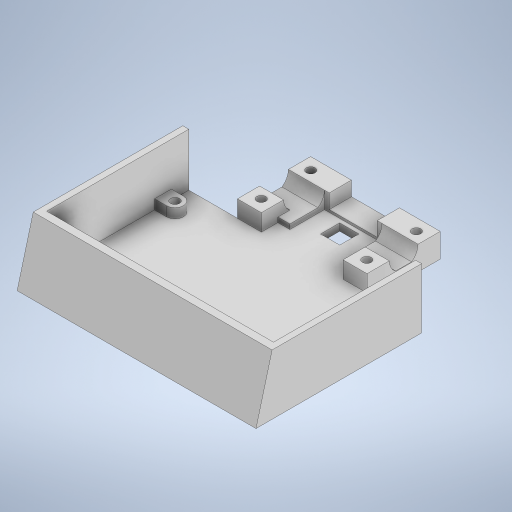
# Autodesk Inventor part: tělo estonsko s plechem otočené motory
Saved by Autodesk Inventor 2024 (Build 280153000, 153)
## iProperties
Created: 2023-09-06
Part Number: tělo estonsko s plechem otočené motory
Material: Všeobecné
Document SubType Name: Modeling
Designer: Simak
Density: 1 g/cm^3
Appearance: Výchozí
Author: Simak
Autodesk Inventor part; units mm, degrees
ref_plane "Pracovní rovina1" through (47.25, 44, 5) normal (0, 1, 0) x (1, 0, 0)
ref_plane "Pracovní rovina2" through (45.625, 37.275, -13.15) normal (0, 1, 0) x (1, 0, 0)
ref_plane "YZ Plane" through (0, 0, 0) normal (1, 0, 0) x (0, 1, 0)
sketch "Náčrt1" plane through (0, 0, 0) normal (0, 1, 0) x (-1, 0, 0)
  line L0 (49.75, -19.25) -> (49.75, 49.75)
  line L1 (49.75, 49.75) -> (-49.75, 49.75)
  line L2 (-49.75, 49.75) -> (-49.75, -19.25)
  line L3 (-49.75, -19.25) -> (-27, -19.25)
  line L4 (-27, -19.25) -> (-27, -49.75)
  line L5 (-27, -49.75) -> (27, -49.75)
  line L6 (27, -49.75) -> (27, -19.25)
  line L7 (27, -19.25) -> (49.75, -19.25)
  point P0 (0, 0)
  dimension "d0" = 30.5
  dimension "d1" = 99.5
  dimension "d2" = 22.75
  dimension "d3" = 99.5
  dimension "d4" = 54
  dimension "d5" = 49.75
  dimension "d6" = 49.75
  constraints: 16 end point, 6 perpendicular, 2 vertical, 1 parallel
  measures "d0" distance of L3.end L4.end
  measures "d1" distance of L0.end L1.end
  measures "d2" distance of L2.end L3.end
  measures "d3" distance between parallel lines of L1 L5
  measures "d4" distance of L4.end L5.end
  measures "d5" horizontal distance of L1.end point (0, 0)
  measures "d6" distance from line of point (0, 0) L1
extrude "Vysunutí1" add sketch "Náčrt1" along normal blind 3
sketch "Náčrt2" plane through (27, 0, -19.25) normal (1, 0, 0) x (0, 0, -1)
  line L0 (30.5, 3) -> (0, 3) projected
  line L1 (0, 3) -> (0, 10)
  line L2 (0, 10) -> (9.2501, 10)
  line L3 (21.2499, 10) -> (30.5, 10)
  line L4 (30.5, 10) -> (30.5, 3)
  line L5 (0, 0) -> (30.5, 0) projected
  line L6 (11.9334, 5) -> (18.5664, 5)
  line L7 (11.9334, 15) -> (18.5664, 15)
  arc A0 (11.9334, 15) -> (11.9334, 5) centre (15.2501, 10) ccw
  arc A1 (18.5664, 5) -> (18.5664, 15) centre (15.2501, 10) ccw
  point P0 (-19.25, 0)
  point P1 (9.2501, 10)
  dimension "d449" = 6.633
  dimension "d450" = 10
  dimension "d452" = 6
  dimension "d453" = 5
  constraints: 12 end point, 6 point on circle, 4 coincident, 2 centre point, 2 equal length, 2 horizontal, 2 perpendicular, 2 point on line, 1 vertical, 1 vertical alignment
  measures "d449" distance of L6.start L6.end
  measures "d450" distance between parallel lines of L7 L6
  measures "d452" radius of A0
  measures "d453" distance between parallel lines of L5 L6
extrude "Vysunutí2" add sketch "Náčrt2" against normal up to surface (54 mm away) contours L0 L1 L2 A0 L6 A1 L3 L4
sketch "Náčrt3" plane through (27, 3, -19.25) normal (0, 0, 1) x (1, 0, 0)
  line L0 (-54, 7) -> (-54, 0) projected
  line L1 (0, -3) -> (-54, -3) projected
  line L2 (-54, -3) -> (-54, 7) projected
  line L3 (0, 7) -> (-54, 7) projected
  line L4 (0, -3) -> (0, 7) projected
  line L5 (-54, 0) -> (0, 0)
  line L6 (-39, 0) -> (-39, 7)
  line L7 (-15, 0) -> (-15, 7)
  line L8 (-39, 3.5) -> (-15, 3.5) construction
  point P0 (-27, -3)
  point P1 (-27, 3.5)
  point P2 (-27, -3)
  dimension "d454" = 24
  constraints: 8 end point, 5 point on line, 4 midpoint, 2 perpendicular, 1 parallel, 1 vertical alignment
  measures "d454" distance between parallel lines of L7 L6
extrude "Vysunutí3" cut sketch "Náčrt3" against normal up to surface (21.2499 mm away) contours L3 L7 L5 L6
sketch "Náčrt4" plane through (-27, 3, -19.25) normal (0, 0, 1) x (1, 0, 0)
  line L0 (15, 2) -> (0, 2) projected
  line L1 (54, 2) -> (39, 2) projected
  line L2 (10, 2) -> (10, 7)
  line L3 (15, 7) -> (0, 7) projected
  line L4 (15, 0) -> (15, 7) projected
  line L5 (39, 7) -> (39, 0) projected
  line L6 (54, 7) -> (39, 7) projected
  line L7 (44, 7) -> (44, 2)
  line L8 (54, 7) -> (54, 0) projected
  line L9 (0, 7) -> (0, 0) projected
  point P0 (27, -3)
  dimension "d455" = 10
  dimension "d456" = 10
  constraints: 4 end point, 4 point on line, 1 perpendicular, 1 vertical
  measures "d455" distance between parallel lines of L8 L7
  measures "d456" distance between parallel lines of L9 L2
extrude "Vysunutí4" cut sketch "Náčrt4" against normal up to surface (18.5664 mm away) contours L0 L2 L3 L4 | L1 L5 L6 L7
sketch "Náčrt5" plane through (-27, 3, -19.25) normal (0, 0, 1) x (1, 0, 0)
  line L0 (10, 2) -> (10, 0)
  line L1 (54, 0) -> (0, 0) projected
  line L2 (44, 2) -> (44, 0)
  line L3 (54, 0) -> (39, 0) projected
  line L4 (-22.75, 0) -> (76.75, 0) projected
  line L5 (15, 2) -> (0, 2) projected
  line L6 (15, 0) -> (15, 7) projected
  line L7 (39, 7) -> (39, 0) projected
  line L8 (54, 2) -> (39, 2) projected
  line L9 (10, 2) -> (10, 7) projected
  line L10 (44, 7) -> (44, 2) projected
  point P0 (27, -3)
  point P1 (44, 0)
  constraints: 4 end point, 4 point on line, 2 collinear, 1 parallel, 1 vertical
extrude "Vysunutí5" cut sketch "Náčrt5" against normal blind 6.875
sketch "Náčrt6" plane through (27, 7.646, -40.4999) normal (0, 0, 1) x (1, 0, 0)
  line L0 (-37, 2.354) -> (-37, -3.646)
  line L1 (-37, -3.646) -> (-17, -3.646)
  line L2 (-17, -3.646) -> (-17, 2.354)
  line L3 (-76.75, -4.646) -> (22.75, -4.646) projected
  line L4 (-54, -7.646) -> (-54, 2.354) projected
  line L5 (-15, 2.354) -> (-39, 2.354) projected
  point P0 (-27, -7.646)
  point P1 (-27, 2.354)
  point P2 (-27, -3.646)
  dimension "d27" = 1
  dimension "d35" = 20
  constraints: 6 end point, 2 midpoint, 2 perpendicular, 2 point on line, 1 vertical, 1 vertical alignment
  measures "d27" distance between parallel lines of L3 L1
  measures "d35" distance of L0.end L1.end
extrude "Vysunutí6" cut sketch "Náčrt6" against normal up to next
sketch "Náčrt7" plane through (-27, 10, -19.25) normal (0, 1, 0) x (1, 0, 0)
  circle A0 centre (5, 4.9375) radius 1.85
  circle A1 centre (5, 25.5625) radius 1.85
  circle A2 centre (49, 25.5625) radius 1.85
  circle A3 centre (49, 4.9375) radius 1.85
  line L0 (76.75, 0) -> (54, 0) projected
  line L1 (49, 4.9375) -> (54, 0) construction
  line L2 (54, 0) -> (44, 0) projected
  line L3 (44, 0) -> (49, 4.9375) construction
  line L4 (54, 9.875) -> (49, 4.9375) construction
  line L5 (10, 0) -> (10, 6.875) projected
  line L6 (5, 4.9375) -> (10, 0) construction
  line L7 (0, 30.5) -> (0, 0) projected
  line L8 (0, 0) -> (5, 4.9375) construction
  line L9 (5, 4.9375) -> (0, 9.875) construction
  line L10 (0, 20.625) -> (5, 25.5625) construction
  line L11 (5, 25.5625) -> (0, 30.5) construction
  line L12 (54, 0) -> (54, 30.5) projected
  line L13 (54, 20.625) -> (49, 25.5625) construction
  line L14 (49, 25.5625) -> (54, 30.5) construction
  dimension "d0" = 30.5
  dimension "d36" = 3.7
  constraints: 20 end point, 12 equal length, 4 centre point, 3 equal radius, 1 coincident
  measures "d36" diameter of A1
extrude "Vysunutí7" cut sketch "Náčrt7" against normal through all
sketch "Náčrt28" plane through (0, 3, 0) normal (0, 1, 0) x (1, 0, 0)
  circle A0 centre (-42.25, 8.5) radius 1.85
  circle A1 centre (42.25, 8.5) radius 1.85
  circle A2 centre (42.25, -29) radius 1.85
  circle A3 centre (-42.25, -29) radius 1.85
  line L0 (-42.25, 8.5) -> (-49.75, 8.5) construction
  line L1 (-49.75, 19.25) -> (-49.75, -49.75) projected
  line L2 (42.25, 8.5) -> (49.75, 8.5) construction
  line L3 (49.75, -49.75) -> (49.75, 19.25) projected
  line L4 (-49.75, -49.75) -> (49.75, -49.75) projected
  point P0 (0, 0)
  dimension "d185" = 3.7
  dimension "d186" = 84.5
  dimension "d187" = 37.5
  dimension "d195" = 20.75
  constraints: 4 centre point, 4 end point, 3 equal radius, 3 point on line, 2 horizontal alignment, 2 vertical alignment, 1 collinear, 1 horizontal
  measures "d185" diameter of A0
  measures "d186" distance of L2.start L0.start
  measures "d187" distance of A3.centre L0.start
  measures "d195" distance from line of L4 A3.centre
sketch "Náčrt29" plane through (49.75, 0, 49.75) normal (1, 0, 0) x (0, 0, -1)
  line L0 (0, 0) -> (69, 0) projected
  line L1 (0, 0) -> (6.6987, 25)
  line L2 (6.6987, 25) -> (9.8046, 25)
  line L3 (9.8046, 25) -> (3.9097, 3)
  line L4 (0, 3) -> (69, 3) projected
  line L5 (0, 0) -> (0, 3) projected
  point P0 (49.75, 0)
  point P1 (0.8038, 3)
  dimension "d188" = 75
  dimension "d189" = 25
  dimension "d190" = 3
  constraints: 6 end point, 1 horizontal, 1 parallel, 1 point on line
  measures "d188" angle of L0 L1
  measures "d189" distance between parallel lines of L0 L2
  measures "d190" distance between parallel lines of L1 L3
extrude "Vysunutí31" add sketch "Náčrt29" against normal up to surface (99.5 mm away) contours L1 L2 L3 L4
extrude "Vysunutí32" cut sketch "Náčrt29" against normal through all contours L5 L4 L1
extrude "Vysunutí33" cut sketch "Náčrt28" against normal up to next
sketch "Náčrt31" plane through (0, 3, 0) normal (0, 1, 0) x (1, 0, 0)
  line L0 (37.136, -36.833) -> (45.136, -36.833)
  line L1 (45.136, -36.833) -> (45.136, -44.833)
  line L2 (45.136, -44.833) -> (37.136, -44.833)
  line L3 (37.136, -44.833) -> (37.136, -36.833)
  line L4 (-4, -36.833) -> (4, -36.833)
  line L5 (4, -36.833) -> (4, -44.833)
  line L6 (4, -44.833) -> (-4, -44.833)
  line L7 (-4, -44.833) -> (-4, -36.833)
  line L8 (-45.463, -36.833) -> (-37.463, -36.833)
  line L9 (-37.463, -36.833) -> (-37.463, -44.833)
  line L10 (-37.463, -44.833) -> (-45.463, -44.833)
  line L11 (-45.463, -44.833) -> (-45.463, -36.833)
  line L12 (49.75, -45.8403) -> (49.75, 19.25) projected
  line L13 (-49.75, 19.25) -> (-49.75, -45.8403) projected
  line L14 (-49.75, -49.75) -> (49.75, -49.75) projected
  line L15 (4, 38.875) -> (-4, 38.875)
  line L16 (-4, 38.875) -> (-4, 30.875)
  line L17 (-4, 30.875) -> (4, 30.875)
  line L18 (4, 30.875) -> (4, 38.875)
  line L19 (4, 34.875) -> (27, 34.875) construction
  line L20 (-4, 34.875) -> (-27, 34.875) construction
  line L21 (-27, 49.75) -> (-27, 19.25) projected
  line L22 (27, 19.25) -> (27, 49.75) projected
  line L23 (10, 40.4999) -> (-10, 40.4999) projected
  point P0 (0, 0)
  point P1 (0, -36.833)
  dimension "d198" = 8
  dimension "d199" = 4.614
  dimension "d200" = 4.287
  dimension "d201" = 4.917
  dimension "d457" = 1.6249
  constraints: 36 end point, 8 equal length, 8 parallel, 6 horizontal, 4 perpendicular, 3 midpoint, 3 point on line, 2 horizontal alignment, 1 vertical alignment
  measures "d198" distance between parallel lines of L2 L0
  measures "d199" distance between parallel lines of L12 L1
  measures "d200" distance between parallel lines of L13 L11
  measures "d201" distance from line of L14 L5.end
  measures "d457" distance between parallel lines of L23 L15
extrude "Vysunutí34" cut sketch "Náčrt31" against normal up to next
sketch "Náčrt32" plane through (-27, 0, -19.25) normal (0, 0, -1) x (-1, 0, 0)
  line L0 (0, 0) -> (22.75, 0) projected
  line L1 (22.75, 0) -> (20.25, 0)
  line L2 (20.25, 0) -> (20.25, 25)
  line L3 (20.25, 25) -> (22.75, 25)
  line L4 (22.75, 25) -> (22.75, 0)
  line L5 (-76.75, 0) -> (-74.25, 0)
  line L6 (-74.25, 0) -> (-74.25, 25)
  line L7 (-74.25, 25) -> (-76.75, 25)
  line L8 (-76.75, 25) -> (-76.75, 0)
  line L9 (-76.75, 25) -> (22.75, 25) projected
  point P0 (-27, 0)
  point P1 (20.25, 0)
  dimension "d204" = 2.5
  constraints: 16 end point, 4 parallel, 2 horizontal, 2 perpendicular, 1 collinear, 1 point on line
  measures "d204" distance between parallel lines of L2 L4
extrude "Vysunutí35" add sketch "Náčrt32" against normal up to next
sketch "Náčrt34" plane through (0, 3, 0) normal (0, 1, 0) x (1, 0, 0)
  circle A0 centre (42.25, -29) radius 1.85 projected
  circle A1 centre (42.25, 8.5) radius 1.85 projected
  circle A2 centre (-42.25, 8.5) radius 1.85 projected
  circle A3 centre (-42.25, -29) radius 1.85 projected
  circle A4 centre (42.25, -29) radius 3.5
  circle A5 centre (42.25, 8.5) radius 3.5
  circle A6 centre (-42.25, 8.5) radius 3.5
  circle A7 centre (-42.25, -29) radius 3.5
  point P0 (0, 0)
  dimension "d214" = 7
  constraints: 4 centre point, 4 coincident, 3 equal radius
  measures "d214" diameter of A4
extrude "Vysunutí37" add sketch "Náčrt34" along normal blind 4
sketch "Náčrt35" plane through (0, 0, 0) normal (0, -1, 0) x (1, 0, 0)
  line L0 (19.175, -25.8185) -> (19.175, -22.5565) projected
  circle A0 centre (42.25, -8.5) radius 1.85 projected
  line L1 (39.425, -10.131) -> (39.425, -6.869)
  line L2 (39.425, -6.869) -> (42.25, -5.238)
  line L3 (42.25, -5.238) -> (45.075, -6.869)
  line L4 (45.075, -6.869) -> (45.075, -10.131)
  line L5 (45.075, -10.131) -> (42.25, -11.762)
  line L6 (42.25, -11.762) -> (39.425, -10.131)
  circle A1 centre (42.25, 29) radius 1.85 projected
  line L7 (39.425, 27.369) -> (39.425, 30.631)
  line L8 (39.425, 30.631) -> (42.25, 32.262)
  line L9 (42.25, 32.262) -> (45.075, 30.631)
  line L10 (45.075, 30.631) -> (45.075, 27.369)
  line L11 (45.075, 27.369) -> (42.25, 25.738)
  line L12 (42.25, 25.738) -> (39.425, 27.369)
  circle A2 centre (-42.25, 29) radius 1.85 projected
  line L13 (-45.075, 27.369) -> (-45.075, 30.631)
  line L14 (-45.075, 30.631) -> (-42.25, 32.262)
  line L15 (-42.25, 32.262) -> (-39.425, 30.631)
  line L16 (-39.425, 30.631) -> (-39.425, 27.369)
  line L17 (-39.425, 27.369) -> (-42.25, 25.738)
  line L18 (-42.25, 25.738) -> (-45.075, 27.369)
  circle A3 centre (-42.25, -8.5) radius 1.85 projected
  line L19 (-45.075, -10.131) -> (-45.075, -6.869)
  line L20 (-45.075, -6.869) -> (-42.25, -5.238)
  line L21 (-42.25, -5.238) -> (-39.425, -6.869)
  line L22 (-39.425, -6.869) -> (-39.425, -10.131)
  line L23 (-39.425, -10.131) -> (-42.25, -11.762)
  line L24 (-42.25, -11.762) -> (-45.075, -10.131)
  point P0 (0, 0)
  constraints: 48 end point, 4 coincident, 4 equal length, 4 vertical, 52 other
extrude "Vysunutí38" [suppressed]
chamfer "Zkosení3" [suppressed]
sketch "Náčrt36" plane through (42.25, 7, -8.5) normal (0, 1, 0) x (1, 0, 0)
  circle A0 centre (0, 0) radius 3.5 projected
  line L0 (0, -3.5) -> (5, -3.5)
  line L1 (5, -54.3403) -> (5, 10.75) projected
  line L2 (0, 3.5) -> (5, 3.5)
  line L3 (0, -34) -> (5, -34)
  circle A1 centre (0, -37.5) radius 3.5 projected
  line L4 (0, -41) -> (5, -41)
  line L5 (-84.5, -41) -> (-89.5, -41)
  line L6 (-89.5, 10.75) -> (-89.5, -54.3403) projected
  circle A2 centre (-84.5, -37.5) radius 3.5 projected
  line L7 (-84.5, -34) -> (-89.5, -34)
  circle A3 centre (-84.5, 0) radius 3.5 projected
  line L8 (-84.5, -3.5) -> (-89.5, -3.5)
  line L9 (-84.5, 3.5) -> (-89.5, 3.5)
  point P0 (-42.25, -8.5)
  point P1 (-84.5, 3.5)
  point P2 (5, 3.5)
  point P3 (0, 3.5)
  dimension "d0" = 30.5
  constraints: 16 end point, 8 horizontal, 6 point on line, 4 perpendicular, 4 tangent, 3 parallel, 3 vertical alignment, 2 point on circle, 4 other
extrude "Vysunutí39" add sketch "Náčrt36" against normal up to next contours A0 L2 L1 L0 | L4 A1 L3 L1 | L5 L6 L7 A2 | L9 A3 L8 L6
sketch "Náčrt37" plane through (27, 7.646, -40.4999) normal (0, 0, 1) x (1, 0, 0)
  line L0 (-15, -4.646) -> (-39, -4.646) projected
  line L1 (-15, 0) -> (-15, -4.646) projected
  line L2 (-39, -4.646) -> (-39, 0) projected
  line L3 (-39, 0) -> (-39, 2.354)
  line L4 (-37, 2.354) -> (-54, 2.354) projected
  line L5 (-15, 0) -> (-15, 2.354)
  line L6 (-15, 2.354) -> (-17.0063, 2.354)
  line L7 (-17.0063, 2.354) -> (-37, 2.354)
  point P0 (-27, -7.646)
  constraints: 8 end point, 2 vertical, 1 collinear, 1 perpendicular, 1 point on line
sketch "Náčrt40" plane through (47.25, 3, -19.25) normal (-1, 0, 0) x (0, 0, 1)
  line L0 (0, -3) -> (0, 22) projected
  line L1 (0, 0) -> (1, 0)
  line L2 (1, 0) -> (1, 10)
  line L3 (1, 10) -> (0, 10)
  line L4 (0, 10) -> (0, 0)
  line L5 (0, 0) -> (7.25, 0) projected
  point P0 (19.25, -3)
  point P1 (0, 10)
  dimension "d236" = 1
  dimension "d237" = 10
  constraints: 8 end point, 2 parallel, 1 horizontal, 1 perpendicular
  measures "d236" distance of L2.end L3.end
  measures "d237" distance between parallel lines of L5 L3
sketch "Náčrt41" plane through (-47.25, 3, -19.25) normal (1, 0, 0) x (0, 0, -1)
  line L0 (-1, 10) -> (0, 10) projected
  line L1 (0, 10) -> (0, 8) projected
  line L2 (0, 0) -> (0, 8) projected
  line L3 (-1, 0) -> (0, 0) projected
  line L4 (-1, 0) -> (-1, 10) projected
  point P0 (-19.25, -3)
sketch "Náčrt44" plane through (-49.75, 25, 43.0513) normal (0, 1, 0) x (1, 0, 0)
  line L0 (97, 3.1058) -> (2.5, 3.1058) projected
  line L1 (32.781, 3.1058) -> (32.781, 11.1058)
  line L2 (24.781, 11.1058) -> (24.781, 3.1058)
  line L3 (0, 62.3013) -> (0, 0) projected
  line L4 (32.781, 11.1058) -> (24.781, 11.1058)
  point P0 (49.75, 43.0513)
  point P1 (0, 18.7254)
  point P2 (28.781, 11.1058)
  dimension "d266" = 8
  dimension "d267" = 28.781
  constraints: 6 end point, 2 perpendicular, 2 point on line, 1 horizontal, 1 midpoint, 1 vertical
  measures "d266" distance between parallel lines of L0 L4
  measures "d267" distance from line of point (28.781, 11.106) L3
sketch "Náčrt46" plane through (-24.969, 25, 31.9454) normal (-1, 0, 0) x (0, 0, 1)
  line L0 (0, -6) -> (8, -6) projected
  line L1 (8, -6) -> (9.6077, -6)
  line L2 (8, 0) -> (13.8949, -22) projected
  line L3 (8, 0) -> (8, -6) projected
  point P0 (-31.9454, -25)
  constraints: 2 end point, 1 horizontal, 1 point on line
sketch "Náčrt45" plane through (-49.75, 25, 43.0513) normal (0, 1, 0) x (1, 0, 0)
  line L0 (32.781, 3.1058) -> (24.781, 3.1058) projected
  line L1 (24.781, 11.1058) -> (24.781, 3.1058) projected
  line L2 (32.781, 11.1058) -> (24.781, 11.1058) projected
  line L3 (99.5, 0) -> (0, 0) projected
  point P0 (49.75, 43.0513)
  point P1 (28.781, 6.196)
  point P2 (28.781, 11.1058)
  dimension "d283" = 6.196
  constraints: 1 midpoint, 1 vertical alignment
  measures "d283" distance from line of point (28.781, 6.196) L3
sketch "Náčrt47" plane through (-16.969, 25, 31.9454) normal (0, 0, -1) x (-1, 0, 0)
  line L0 (1.2, -1.4) -> (6.8, -1.4)
  line L1 (6.8, -1.4) -> (6.8, -4.6)
  line L2 (6.8, -4.6) -> (1.2, -4.6)
  line L3 (1.2, -4.6) -> (1.2, -1.4)
  line L4 (0, 0) -> (8, 0) projected
  line L5 (0, 0) -> (0, -6) projected
  point P0 (-16.969, -25)
  point P1 (4, -1.4)
  point P2 (4, 0)
  point P3 (0, -3)
  point P4 (1.2, -3)
  dimension "d279" = 5.6
  dimension "d280" = 3.2
  constraints: 8 end point, 4 midpoint, 2 parallel, 1 horizontal, 1 horizontal alignment, 1 perpendicular, 1 vertical alignment
  measures "d279" distance of L1.end L2.end
  measures "d280" distance of L0.end L1.end
sketch "Náčrt48" plane through (-49.75, 0, -19.25) normal (-1, 0, 0) x (0, 0, 1)
  line L0 (0, 25) -> (62.3013, 25) projected
  line L1 (0, 25) -> (24.25, 44)
  line L2 (24.25, 44) -> (24.25, 25)
  line L3 (0, 25) -> (62.3013, 25) projected
  point P0 (19.25, 0)
  dimension "d285" = 24.25
  dimension "d286" = 19
  dimension "d289" = 3.2
  dimension "d290" = 5.2
  dimension "d291" = 2
  dimension "d292" = 2
  dimension "d293" = 2
  constraints: 18 end point, 3 perpendicular, 2 collinear, 2 horizontal, 2 midpoint, 2 parallel, 1 point on line, 1 vertical, 1 vertical alignment
  measures "d289" distance of L2.end L3.end
  measures "d290" distance of L1.end L2.end
sketch "Náčrt33" plane through (-49.75, 0, -19.25) normal (-1, 0, 0) x (0, 0, 1)
  line L0 (36.318, 10.36) -> (42.098, 10.36) construction
  line L1 (36.318, 8.78) -> (42.098, 8.78)
  line L2 (42.098, 11.94) -> (36.318, 11.94)
  arc A0 (36.318, 11.94) -> (36.318, 8.78) centre (36.318, 10.36) ccw
  arc A1 (42.098, 8.78) -> (42.098, 11.94) centre (42.098, 10.36) ccw
  line L3 (0, 0) -> (69, 0) projected
  line L4 (0, 0) -> (0, 25) projected
  line L5 (36.318, 14.44) -> (42.098, 14.44)
  arc A2 (42.098, 6.28) -> (42.098, 14.44) centre (42.098, 10.36) ccw
  line L6 (42.098, 6.28) -> (36.318, 6.28)
  arc A3 (36.318, 14.44) -> (36.318, 6.28) centre (36.318, 10.36) ccw
  point P0 (19.25, 0)
  point P1 (39.208, 10.36)
  point P2 (34.738, 10.36)
  point P3 (43.678, 10.36)
  dimension "d207" = 8.78
  dimension "d208" = 3.16
  dimension "d209" = 8.94
  dimension "d210" = 34.738
  dimension "d211" = 2.5
  constraints: 12 end point, 10 point on circle, 4 centre point, 4 tangent, 2 parallel, 1 horizontal, 1 midpoint, 3 other
  measures "d207" distance between parallel lines of L3 L1
  measures "d208" distance between parallel lines of L1 L2
  measures "d209" distance of point (34.738, 10.36) point (43.678, 10.36)
  measures "d210" distance from line of L4 point (34.738, 10.36)
  measures "d211" distance between parallel lines of L2 L5
sketch "Náčrt50" plane through (-27, 0, -49.75) normal (-1, 0, 0) x (0, 0, 1)
  line L0 (0, 0) -> (0, 10) projected
  line L1 (0, 0) -> (30.5, 0) projected
  line L2 (0, 10) -> (0, 3) projected
  line L3 (0, 5.5) -> (10, 0)
  line L4 (0, 6.5) -> (3, 3.85)
  point P0 (49.75, 0)
  point P1 (0, 5.5)
  point P2 (0, 6.5)
  dimension "d316" = 5.5
  dimension "d317" = 10
  dimension "d318" = 6.5
  dimension "d319" = 3
  constraints: 4 end point, 3 point on line, 1 midpoint
  measures "d316" distance of L0.start L3.start
  measures "d317" distance of L0.start L3.end
  measures "d318" distance of L0.start L4.start
  measures "d319" distance from line of L0 L4.end
sketch "Náčrt51" plane through (12, 7.646, -39.875) normal (-1, 0, 0) x (0, 0, -1)
  line L0 (9.875, -3.354) -> (0, -3.354) projected
  line L1 (9.875, 3.354) -> (0, 3.354)
  line L2 (0, 3.354) -> (0, -4.646)
  line L3 (-9.875, -1.146) -> (-9.875, -3.354)
  line L4 (-6.875, -3.796) -> (-5.3295, -4.646) projected
  line L5 (-9.875, -1.146) -> (-6.875, -3.796) projected
  line L6 (13.75, -4.646) -> (-5.3295, -4.646) projected
  point P0 (-39.875, 7.646)
  point P1 (-9.875, -1.146)
  constraints: 6 end point, 2 point on line, 1 coincident, 1 horizontal, 1 parallel, 1 perpendicular
sketch "Náčrt52" plane through (27, 10, -39.875) normal (0, 1, 0) x (1, 0, 0)
  line L0 (-15, 0) -> (-39, 0) projected
  line L1 (0, 9.875) -> (-54, 9.875) projected
  line L2 (-22, 0) -> (-32, 0)
  line L3 (-32, 0) -> (-32, 9.875)
  line L4 (-32, 9.875) -> (-22, 9.875)
  line L5 (-22, 9.875) -> (-22, 0)
  line L6 (-32, 4.9375) -> (-54, 4.9375) construction
  line L7 (-54, 6.875) -> (-54, -0.125) projected
  line L8 (-22, 4.9375) -> (0, 4.9375) construction
  line L9 (0, 9.875) -> (0, 0.6249) projected
  point P0 (-27, -39.875)
  point P1 (0, 0)
  point P2 (-22, 9.875)
  point P3 (-32, 0)
  dimension "d323" = 10
  dimension "d328" = 3.7
  dimension "d389" = 5.65
  constraints: 16 end point, 2 midpoint, 1 centre point, 1 coincident, 1 collinear, 1 vertical, 1 vertical alignment, 13 other
  measures "d389" distance between parallel lines of L8 L5
sketch "Náčrt54" plane through (27, 11, -39.875) normal (0, 1, 0) x (1, 0, 0)
  line L0 (-22, 0) -> (-23, 0)
  line L1 (-23, 0) -> (-23, 9.875)
  line L2 (-23, 9.875) -> (-22, 9.875)
  line L3 (-22, 9.875) -> (-22, 0)
  line L4 (-32, 0) -> (-31, 0)
  line L5 (-31, 0) -> (-31, 9.875)
  line L6 (-31, 9.875) -> (-32, 9.875)
  line L7 (-32, 9.875) -> (-32, 0)
  line L8 (-22, 9.875) -> (-32, 9.875) projected
  line L9 (-32, 0) -> (-22, 0) projected
  line L10 (-22, 0) -> (-22, 9.875) projected
  line L11 (-32, 9.875) -> (-32, 0) projected
  point P0 (-27, -39.875)
  dimension "d331" = 1
  constraints: 16 end point, 7 collinear, 4 parallel, 2 horizontal, 2 perpendicular
  measures "d331" distance of L5.end L6.end
sketch "Náčrt56" plane through (0, 0, 0) normal (0, -1, 0) x (1, 0, 0)
  line L0 (27, -19.25) -> (27, -39.75) projected
  line L1 (49.75, -19.25) -> (27, -19.25) projected
  line L2 (49.75, 49.75) -> (49.75, -19.25) projected
  line L3 (-49.75, 49.75) -> (49.75, 49.75) projected
  line L4 (-49.75, -19.25) -> (-49.75, 49.75) projected
  line L5 (-27, -19.25) -> (-49.75, -19.25) projected
  line L6 (-27, -39.75) -> (-27, -19.25) projected
  line L7 (27, -49.75) -> (-27, -49.75) projected
  line L8 (27, -39.75) -> (27, -46.75) projected
  line L9 (27, -46.75) -> (27, -49.75) projected
  line L10 (-27, -49.75) -> (-27, -46.75) projected
  line L11 (-27, -46.75) -> (-27, -39.75) projected
sketch "Náčrt57" plane through (0, 7, 0) normal (0, 1, 0) x (1, 0, 0)
  arc A0 (-42.25, 5) -> (-42.25, 12) centre (-42.25, 8.5) ccw projected
  line L0 (-47.25, 18.25) -> (-17, 18.25) projected
  arc A1 (-31.5, 15.75) -> (-38.75, 8.5) centre (-31.5, 8.5) ccw
  line L1 (-47.25, -32.5) -> (-47.25, 12) projected
  line L2 (-42.25, 12) -> (-47.25, 12) projected
  arc A2 (42.25, 12) -> (42.25, 5) centre (42.25, 8.5) ccw projected
  line L3 (47.25, 12) -> (42.25, 12) projected
  line L4 (47.25, 12) -> (47.25, 19.25) projected
  line L5 (47.25, 18.25) -> (17, 18.25) projected
  arc A3 (38.75, 8.5) -> (31.5, 15.75) centre (31.5, 8.5) ccw
  line L6 (-47.25, 15.75) -> (-14.5, 15.75)
  line L7 (-49.75, -5) -> (-49.75, 19.25) projected
  line L8 (47.25, 15.75) -> (14.5, 15.75)
  line L9 (-14.5, 15.75) -> (-17, 18.25)
  line L10 (17, 18.25) -> (14.5, 15.75)
  point P0 (0, 0)
  point P1 (-25.25, 18.25)
  point P2 (25.25, 18.25)
  point P3 (29, 18.25)
  point P4 (38.75, 8.5)
  point P5 (-38.75, 8.5)
  point P6 (-29, 18.25)
  dimension "d377" = 2.5
  dimension "d378" = 2.5
  constraints: 8 end point, 6 point on circle, 5 point on line, 3 tangent, 2 centre point, 2 horizontal alignment, 1 collinear, 1 equal radius, 1 horizontal, 1 perpendicular
  measures "d377" distance between parallel lines of L0 L6
  measures "d378" horizontal distance of L8.end L5.end
sketch "Náčrt59" plane through (27, 12, -39.875) normal (0, 1, 0) x (1, 0, 0)
  line L0 (0, 0) -> (-22, 0) projected
  line L1 (-32, 0) -> (-32, 9.875) projected
  line L2 (-22, 0) -> (-32, 0)
  line L3 (-32, 0) -> (-32, 1.5)
  line L4 (-32, 1.5) -> (-22, 1.5)
  line L5 (-22, 1.5) -> (-22, 0)
  line L6 (-22, 0) -> (-22, 9.875) projected
  point P0 (-27, -39.875)
  dimension "d386" = 1.5
  constraints: 8 end point, 3 point on line, 2 parallel, 1 horizontal, 1 perpendicular
  measures "d386" distance of L4.end L2.start
sketch "Náčrt60" plane through (0, 3, 0) normal (0, -1, 0) x (1, 0, 0)
  arc A0 (23.808, -45.2045) -> (20.192, -45.2045) centre (22, -44.8125) ccw projected
  arc A1 (-20.192, -45.2045) -> (-23.808, -45.2045) centre (-22, -44.8125) ccw projected
  point P0 (0, 0)
  point P1 (22, -44.8125)
  point P2 (-22, -44.8125)
  constraints: 2 coincident
sketch "Náčrt61" plane through (22, 8, -44.8125) normal (0, -1, 0) x (1, 0, 0)
  circle A0 centre (0, 0) radius 1.85 projected
  circle A1 centre (-44, 0) radius 1.85 projected
  point P0 (-22, 44.8125)
  point P1 (0, 0)
  point P2 (-44, 0)
  constraints: 2 coincident
sketch "Náčrt62" plane through (47.25, 44, 5) normal (0, 1, 0) x (1, 0, 0)
  line L0 (0, 12.2) -> (0, 0) projected
  line L1 (0, 2) -> (-6.75, 2)
  line L2 (0, 0) -> (-3.95, 0) projected
  line L3 (0, 0) -> (-6.75, 0)
  line L4 (-6.75, 0) -> (-6.75, 2)
  line L5 (2.5, 0) -> (2.5, 24.25) projected
  line L6 (2.5, 0) -> (0, 0) projected
  line L7 (0, 2) -> (2.5, 2)
  point P0 (-47.25, 5)
  dimension "d404" = 2
  dimension "d405" = 6.75
  dimension "d408" = 12.65
  dimension "d413" = 3.5
  dimension "d414" = 3.5
  dimension "d415" = 2.75
  constraints: 8 end point, 2 point on circle, 2 point on line, 2 tangent, 1 centre point, 1 equal length, 1 perpendicular, 1 vertical
  measures "d415" distance from line of L0 L1.end
sketch "Náčrt65" plane through (49.75, 44, -13.15) normal (0, 0, -1) x (-1, 0, 0)
  line L0 (9.25, 0) -> (9.25, -1.6) projected
  line L1 (9.25, -1.6) -> (2.5, -8.35)
  line L2 (2.5, -11.8) -> (2.5, -1.6) projected
  line L3 (9.25, -1.6) -> (2.5, -1.6) projected
  point P0 (49.75, -44)
  dimension "d416" = 45
  constraints: 2 end point, 1 point on line
  measures "d416" angle of L2 L1
sketch "Náčrt66" plane through (45.3, 32.2, 5) normal (0, 0, 1) x (1, 0, 0)
  line L0 (1.95, 3.45) -> (-4.8, 10.2) projected
  line L1 (1.95, 10.2) -> (-4.8, 10.2) projected
  line L2 (1.95, 0) -> (1.95, 10.2) projected
  point P0 (-45.3, -32.2)
  dimension "d423" = 5.25
  constraints: 12 end point, 2 coincident, 1 horizontal alignment, 16 other
sketch "Náčrt69" plane through (47.25, 44, 5) normal (0, 1, 0) x (1, 0, 0)
  line L0 (0, 0) -> (-3.95, 0) projected
  line L1 (-2.2, 0) -> (-2.2, 0.8)
  arc A0 (-2.2, 0.8) -> (-4.6, 0.8) centre (-3.4, 0.8) ccw
  line L2 (-4.6, 0.8) -> (-4.6, 0)
  line L3 (0, 14.65) -> (0, 2) projected
  line L4 (0, 2) -> (-6.75, 2) projected
  line L5 (-6.75, 0) -> (2.5, 0) projected
  point P0 (-47.25, 5)
  dimension "d428" = 2.2
  dimension "d429" = 1.2
  constraints: 4 end point, 3 tangent, 2 point on circle, 2 point on line, 1 centre point, 1 parallel, 1 vertical
  measures "d428" distance between parallel lines of L3 L1
  measures "d429" radius of A0
sketch "Náčrt70" plane through (45.3, 25, -5.2) normal (0, 0, 1) x (1, 0, 0)
  line L0 (0, 0) -> (0, 3.4) projected
  line L1 (1.8, 5.2) -> (0, 3.4) projected
  line L2 (1.8, 5.2) -> (3.2, 5.2) projected
  line L3 (3.2, 5.2) -> (3.2, 0) projected
  line L4 (0, 0) -> (3.2, 0) projected
  point P0 (-45.3, -25)
